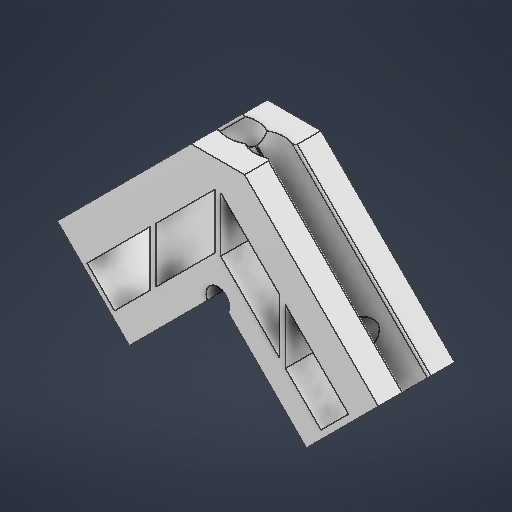
# Autodesk Inventor part: ESCUADRA UNIÓN 45 DISEÑO NUEVO
Saved by Autodesk Inventor 2025 (Build 290162000, 162)
## iProperties
Created: 2026-02-04
Part Number: ESCUADRA UNIÓN 45 DISEÑO NUEVO
Material: Aluminio
Document SubType Name: Modeling
Designer: Frank
Density: 2.7 g/cm^3
Appearance: Satinado
Author: Frank
Autodesk Inventor part; units mm, degrees
note: some values were not read from the file. Chosen so that the rebuilt part matches the saved one: direction of "Agujero1".
sketch "Sketch1" plane through (0, 0, 0) normal (0, 0, 1) x (1, 0, 0)
  line L0 (-0.8, 10.8409) -> (-0.8, 25.973)
  line L1 (-7.3761, 33.539) -> (7.3761, 33.539)
  line L2 (-7.3761, 33.539) -> (-44.1456, -3.2305)
  line L3 (-44.1456, -3.2305) -> (-24.3467, -23.0295)
  line L4 (-24.3467, -23.0295) -> (-2.8506, -1.5335)
  line L5 (0, 40.4641) -> (0, -16.545) construction
  arc A0 (2.8506, -1.5335) -> (-2.8506, -1.5335) centre (0, 0) ccw
  line L6 (-18.6, 8.173) -> (-35.9432, -9.1702)
  line L7 (-35.9432, -9.1702) -> (-28.3772, -16.7362)
  line L8 (-17, 9.773) -> (-17, -5.3591)
  line L9 (-18.6, 8.173) -> (-18.6, -6.9591)
  line L10 (-0.8, 25.973) -> (-17, 9.773)
  line L11 (-28.3772, -16.7362) -> (-18.6, -6.9591)
  line L12 (-17, -5.3591) -> (-0.8, 10.8409)
  line L13 (0.8, 10.8409) -> (0.8, 25.973)
  line L14 (7.3761, 33.539) -> (44.1456, -3.2305)
  line L15 (44.1456, -3.2305) -> (24.3467, -23.0295)
  line L16 (24.3467, -23.0295) -> (2.8506, -1.5335)
  line L17 (18.6, 8.173) -> (35.9432, -9.1702)
  line L18 (35.9432, -9.1702) -> (28.3772, -16.7362)
  line L19 (17, 9.773) -> (17, -5.3591)
  line L20 (18.6, 8.173) -> (18.6, -6.9591)
  line L21 (0.8, 25.973) -> (17, 9.773)
  line L22 (28.3772, -16.7362) -> (18.6, -6.9591)
  line L23 (17, -5.3591) -> (0.8, 10.8409)
  point P0 (0, 33.539)
  dimension "d72" = 30.4
  dimension "d74" = 28
  dimension "d102" = 1.6
  dimension "d106" = 0.8
  dimension "d111" = 33.5
  dimension "d112" = 52
  dimension "d113" = 45
  dimension "d115" = 10
  dimension "d116" = 39
  dimension "d117" = 1.6
  dimension "d135" = 17
  dimension "d139" = 1.6
  dimension "d195" = 3.2369
  dimension "d196" = 7.3
  constraints: 48 end point, 13 symmetric about line, 5 parallel, 5 point on line, 3 vertical, 2 collinear, 2 point on circle, 1 centre point, 1 coincident, 1 horizontal, 1 midpoint, 1 perpendicular
  measures "d72" distance of L4.end L3.end
  measures "d74" distance of L2.end L3.end
  measures "d102" distance between parallel lines of L7 L3
  measures "d106" distance between parallel lines of L0 L5
  measures "d111" distance from line of L3 point (0, 0)
  measures "d112" distance of L1.start L2.end
  measures "d113" angle of L2 L0
  measures "d115" distance between parallel lines of L2 L6
  measures "d116" distance of L0.start L11.start
  measures "d117" distance between parallel lines of L9 L8
  measures "d135" distance between parallel lines of L8 L5
  measures "d139" distance between parallel lines of L0 L13
  measures "d195" radius of A0
  measures "d196" distance between parallel lines of L4 L11
extrude "Extrusion1" add sketch "Sketch1" against normal blind 21
sketch "Boceto2" plane through (24.3467, -23.0295, 0) normal (0.7071068, -0.7071068, 0) x (-0.7071068, -0.7071068, 0)
  line L0 (-35.1512, 10.5) -> (2.0426, 10.5) construction
  line L1 (-28, 21) -> (0, 21) projected
  line L2 (0, 0) -> (-28, 0) projected
  line L3 (-28, 0) -> (-28, 21) projected
  arc A0 (-6.6379, 10.25) -> (0, 7.5) centre (-2.6458, 10.5) ccw
  arc A1 (0, 13.5) -> (-6.6379, 10.75) centre (-2.6458, 10.5) ccw
  line L4 (0, 7.5) -> (0, 13.5)
  line L5 (0, 0) -> (0, 21) projected
  line L6 (-7.1379, 10.25) -> (-7.1379, 10.75)
  line L7 (-7.1379, 10.75) -> (-6.6379, 10.75)
  line L8 (-7.1379, 10.25) -> (-6.6379, 10.25)
  point P0 (0.9314, 0)
  dimension "d142" = 10.5
  dimension "d143" = 10.5
  dimension "d153" = 6
  dimension "d154" = 3
  dimension "d155" = 4
  dimension "d176" = 0.25
  dimension "d177" = 0.5
  dimension "d178" = 0.5
  constraints: 11 end point, 4 point on circle, 2 centre point, 2 horizontal, 2 perpendicular, 1 collinear, 1 point on line
  measures "d142" distance between parallel lines of L0 L2
  measures "d143" distance between parallel lines of L1 L0
  measures "d153" distance of L4.end L4.start
  measures "d154" distance from line of L4.start L0
  measures "d155" radius of A1
  measures "d176" distance between parallel lines of L0 L8
  measures "d177" distance between parallel lines of L8 L7
  measures "d178" distance of L6.end L7.end
extrude "Extrusión2" cut sketch "Boceto2" against normal blind 40.5 contours L4 A0 L8 L6 L7 A1
ref_plane "Plano de trabajo5" through (0, 10.8409, 0) normal (1, 0, 0) x (0, 0, -1)
mirror "Simetría4" about plane through (0, 10.8409, 0) normal (1, 0, 0) of "Extrusión2"
ref_plane "Plano de trabajo7" through (44.1456, -3.2305, -21) normal (0.7071068, 0.7071068, 0) x (-0.7071068, 0.7071068, 0)
sketch "Boceto3" plane through (44.1456, -3.2305, 0) normal (0.7071068, -0.7071068, 0) x (-0.7071068, -0.7071068, 0)
  line L0 (-3.8291, 10.5) -> (9.1738, 10.5) construction
  line L1 (0, 7.5) -> (0, 13.5)
  arc A0 (0, 7.5) -> (6.6379, 10.25) centre (2.6458, 10.5) ccw
  arc A1 (6.6379, 10.75) -> (0, 13.5) centre (2.6458, 10.5) ccw
  line L2 (0, 21) -> (28, 21) projected
  line L3 (28, 0) -> (0, 0) projected
  line L4 (7.1379, 10.75) -> (7.1379, 10.25)
  line L5 (7.1379, 10.25) -> (6.6379, 10.25)
  line L6 (7.1379, 10.75) -> (6.6379, 10.75)
  point P0 (0.9314, 0)
  dimension "d163" = 6
  dimension "d164" = 3
  dimension "d167" = 4
  dimension "d171" = 10.5
  dimension "d172" = 10.5
  dimension "d179" = 0.25
  dimension "d180" = 0.5
  dimension "d181" = 0.5
  constraints: 10 end point, 4 point on circle, 3 horizontal, 2 centre point, 1 vertical
  measures "d163" distance of L1.end L1.start
  measures "d164" distance from line of L1.start L0
  measures "d167" radius of A1
  measures "d171" distance between parallel lines of L2 L0
  measures "d172" distance between parallel lines of L3 L0
  measures "d179" distance between parallel lines of L0 L6
  measures "d180" distance between parallel lines of L6 L5
  measures "d181" distance of L4.end L5.end
extrude "Extrusión3" cut sketch "Boceto3" against normal through all
mirror "Simetría5" about plane through (0, 10.8409, 0) normal (1, 0, 0) of "Extrusión3"
fillet "Empalme1" radius 0.5 8 edges at (13.5986, -12.2815, -13.5) (13.5986, -12.2815, -7.5) (25.7609, 15.1543, -7.5) (25.7609, 15.1543, -13.5) (-25.7609, 15.1543, -13.5) (-25.7609, 15.1543, -7.5) (-13.5986, -12.2815, -7.5) (-13.5986, -12.2815, -13.5)
ref_plane "Plano de trabajo6" through (0, 0, -10.5) normal (0, 0, 1) x (1, 0, 0)
sketch "Boceto7" plane through (44.1456, -3.2305, -21) normal (0.7071068, 0.7071068, 0) x (-0.7071068, 0.7071068, 0)
  arc A0 (52, 14.4555) -> (52.7384, 14.016) centre (52.5, 14.4555) ccw projected
  line L0 (52, 14.4555) -> (0, 14.4555) projected
  line L1 (0, 14.4555) -> (0, 14.016) projected
  line L2 (0, 14.016) -> (52.7384, 14.016) projected
  line L3 (0, 14.016) -> (52.7384, 14.016) projected
  line L4 (0, 10.75) -> (0, 14.016) projected
  line L5 (0, 10.75) -> (55.7934, 10.75) projected
  arc A1 (57.2157, 13.5652) -> (55.7934, 10.75) centre (59.7856, 10.5) ccw projected
  arc A2 (57.2157, 13.5652) -> (52.7384, 14.016) centre (54.6458, 10.5) ccw projected
  line L6 (0, 10.75) -> (55.7934, 10.75) projected
  line L7 (0, 10.75) -> (55.2934, 10.75) projected
  line L8 (55.7934, 10.75) -> (55.2934, 10.75) projected
  line L9 (55.2934, 10.25) -> (55.2934, 10.75) projected
  line L10 (0, 10.75) -> (55.2934, 10.75) projected
  line L11 (0, 10.25) -> (0, 10.75) projected
  line L12 (0, 10.25) -> (55.2934, 10.25) projected
  line L13 (0, 10.25) -> (55.2934, 10.25) projected
  line L14 (0, 10.25) -> (55.7934, 10.25) projected
  line L15 (55.2934, 10.25) -> (55.7934, 10.25) projected
  line L16 (52.7384, 6.984) -> (0, 6.984) projected
  arc A3 (52.7384, 6.984) -> (57.2157, 7.4348) centre (54.6458, 10.5) ccw projected
  arc A4 (55.7934, 10.25) -> (57.2157, 7.4348) centre (59.7856, 10.5) ccw projected
  line L17 (0, 10.25) -> (55.7934, 10.25) projected
  line L18 (0, 6.984) -> (0, 10.25) projected
  line L19 (0, 6.984) -> (0, 6.5445) projected
  line L20 (0, 6.5445) -> (52, 6.5445) projected
  arc A5 (52.7384, 6.984) -> (52, 6.5445) centre (52.5, 6.5445) ccw projected
  line L21 (52.7384, 6.984) -> (0, 6.984) projected
  line L22 (0, 6.5445) -> (52, 6.5445) projected
  line L23 (0, 6.5445) -> (0, 0) projected
  line L24 (52, 0) -> (0, 0) projected
  line L25 (52, 6.5445) -> (52, 0) projected
  line L26 (52, 14.4555) -> (0, 14.4555) projected
  line L27 (52, 21) -> (52, 14.4555) projected
  line L28 (0, 21) -> (52, 21) projected
  line L29 (0, 21) -> (0, 14.4555) projected
  circle A6 centre (14, 10.5) radius 3
  point P0 (33.5, 21)
  dimension "d183" = 6
  dimension "d184" = 10.5
  dimension "d185" = 10.5
  dimension "d186" = 14
  constraints: 1 centre point
  measures "d183" diameter of A6
  measures "d184" distance from line of L24 A6.centre
  measures "d185" distance from line of L28 A6.centre
  measures "d186" distance from line of L23 A6.centre
hole "Agujero1" at (34.2462, 6.669, -10.5) direction (-0.7071068, -0.7071068, 0) diameter 6 depth 10
mirror "Simetría6" about plane through (0, 10.8409, 0) normal (1, 0, 0) of "Agujero1"
thread "Rosca4" size "M6x1" class "6H" standard "ANSI Metric M Profile" full length
thread "Rosca5" size "M6x1" class "6H" standard "ANSI Metric M Profile" full length
body "Solid1"
